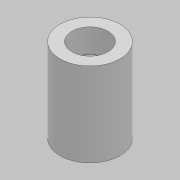
# Autodesk Inventor part: exercise1-2
Saved by Autodesk Inventor 2018 (Build 220112000, 112)
## iProperties
Created: 2020-09-19
Part Number: exercise1-2
Material: 一般
Document SubType Name: Modeling
Designer: 王鼎鈞
Density: 1 g/cm^3
Appearance: 預設
Author: 王鼎鈞
Autodesk Inventor part; units mm, degrees
ref_plane "YZ Plane" through (0, 0, 0) normal (1, 0, 0) x (0, 1, 0)
ref_plane "XZ Plane" through (0, 0, 0) normal (0, 1, 0) x (-1, 0, 0)
ref_plane "XY Plane" through (0, 0, 0) normal (0, 0, 1) x (1, 0, 0)
sketch "草圖1" plane through (0, 0, 0) normal (1, 0, 0) x (0, 1, 0)
  line L0 (-10, 0) -> (60, 0) projected
  line L1 (0, -168) -> (0, 28) projected
  line L2 (0, 0) -> (50, 0)
  line L3 (50, 0) -> (50, -140)
  line L4 (50, -140) -> (0, -140)
  line L5 (0, -140) -> (0, 0)
  line L6 (0, 0) -> (30, 0)
  line L7 (30, 0) -> (30, -40)
  line L8 (30, -40) -> (0, -40)
  line L9 (0, -40) -> (0, 0)
  line L10 (0, -40) -> (10, -40)
  line L11 (10, -40) -> (10, -120)
  line L12 (10, -120) -> (0, -120)
  line L13 (0, -120) -> (0, -40)
  dimension "d0" = 50
  dimension "d1" = 140
  dimension "d2" = 40
  dimension "d3" = 120
  dimension "d4" = 30
  dimension "d5" = 10
  constraints: 24 end point, 6 parallel, 3 horizontal, 3 perpendicular
  measures "d0" distance of L3.end L4.end
  measures "d1" distance of L2.end L3.end
  measures "d2" distance of L6.end L7.end
  measures "d3" distance between parallel lines of L0 L12
  measures "d4" distance of L7.end L8.end
  measures "d5" distance of L11.end L12.end
revolve "迴轉1" add sketch "草圖1" angle 360 about axis through (0, 0, -140) along (0, 0, 1) contours L0 L3 L4 L1 L12 L11 L8 L7
